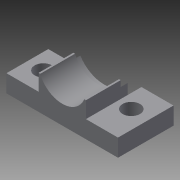
# Autodesk Inventor part: Gbase 3
Saved by Autodesk Inventor 2013 (Build 170138000, 138)
## iProperties
Created: 2016-06-22
Part Number: Gbase 3
Material: Generic
Document SubType Name: Modeling
Designer: labuser
Density: 1 g/cm^3
Author: labuser
Autodesk Inventor part; units mm, degrees
ref_plane "YZ Plane" through (0, 0, 0) normal (1, 0, 0) x (0, 1, 0)
ref_plane "XZ Plane" through (0, 0, 0) normal (0, 1, 0) x (-1, 0, 0)
ref_plane "XY Plane" through (0, 0, 0) normal (0, 0, 1) x (1, 0, 0)
sketch "Sketch1" plane through (0, 0, 0) normal (0, 1, 0) x (-1, 0, 0)
  line L0 (0, 0) -> (20.32, 0)
  line L1 (20.32, 0) -> (20.32, 7.62)
  line L2 (20.32, 7.62) -> (0, 7.62)
  line L3 (0, 7.62) -> (0, 0)
  dimension "d0" = 20.32
  dimension "d1" = 7.62
  constraints: 8 end point, 2 parallel, 1 horizontal, 1 perpendicular
  measures "d0" distance of L2.end L1.end
  measures "d1" distance of L1.end L0.end
extrude "Extrusion1" add sketch "Sketch1" along normal blind 3.175
sketch "Sketch2" plane through (0, 3.175, 0) normal (0, 1, 0) x (1, 0, 0)
  line L0 (0, 0) -> (-20.32, 0) projected
  line L1 (-20.32, 0) -> (-20.32, -7.62) projected
  line L2 (-20.32, -7.62) -> (0, -7.62) projected
  line L3 (-14.478, -7.62) -> (-5.842, -7.62)
  line L4 (-5.842, -7.62) -> (-5.842, 0)
  line L5 (-5.842, 0) -> (-14.478, 0)
  line L6 (-14.478, 0) -> (-14.478, -7.62)
  dimension "d4" = 8.636
  dimension "d5" = 5.842
  constraints: 8 end point, 2 parallel, 2 point on line, 1 horizontal, 1 perpendicular
  measures "d4" distance of L5.end L4.end
  measures "d5" distance between parallel lines of L6 L1
extrude "Extrusion2" add sketch "Sketch2" along normal blind 7.112 contours L4 L2 L6 L0
sketch "Sketch3" plane through (-20.32, 0, 7.62) normal (0, 0, 1) x (1, 0, 0)
  line L0 (14.478, 3.175) -> (14.478, 10.287) projected
  line L1 (5.842, 10.287) -> (14.478, 10.287) projected
  circle A0 centre (10.16, 7.747) radius 4.318
  line L2 (5.842, 10.287) -> (14.478, 10.287)
  line L3 (14.478, 10.287) -> (14.478, 7.747)
  line L4 (14.478, 7.747) -> (5.842, 7.747)
  line L5 (5.842, 7.747) -> (5.842, 10.287)
  line L6 (5.842, 7.747) -> (14.478, 7.747)
  line L7 (14.478, 7.747) -> (14.478, 6.1492)
  line L8 (14.478, 6.1492) -> (5.842, 6.1492)
  line L9 (5.842, 6.1492) -> (5.842, 7.747)
  dimension "d8" = 8.636
  dimension "d9" = 2.54
  constraints: 16 end point, 4 parallel, 2 horizontal, 2 perpendicular, 2 point on line, 1 horizontal alignment, 2 other
  measures "d9" distance from line of L1 point (10.16, 7.747)
extrude "Extrusion3" cut sketch "Sketch3" against normal up to surface (7.62 mm away)
sketch "Sketch5" plane through (0, 0, 0) normal (0, 0, -1) x (-1, 0, 0)
  arc A0 (6.1485, 6.1492) -> (14.1715, 6.1492) centre (10.16, 7.747) ccw projected
  circle A1 centre (10.16, 7.747) radius 5.08
  dimension "d21" = 10.16
  constraints: 1 centre point, 1 coincident
  measures "d21" diameter of A1
extrude "Extrusion5" cut sketch "Sketch5" against normal blind 1.27
sketch "Sketch4" plane through (0, 0, 0) normal (0, -1, 0) x (1, 0, 0)
  line L0 (-20.32, 7.62) -> (0, 7.62) projected
  line L1 (-20.32, 0) -> (-20.32, 7.62) projected
  circle A0 centre (-17.399, 3.81) radius 1.5875
  circle A1 centre (-3.302, 1.8923) radius 1.5875
  dimension "d12" = 3.175
  dimension "d14" = 3.81
  dimension "d15" = 2.921
  dimension "d16" = 3.175
  dimension "d26" = 14.097
  dimension "d27" = 1.9177
  constraints: 2 centre point
  measures "d12" diameter of A0
  measures "d14" distance from line of L0 A0.centre
  measures "d15" distance from line of L1 A0.centre
  measures "d16" diameter of A1
  measures "d26" horizontal distance of A0.centre A1.centre
  measures "d27" vertical distance of A0.centre A1.centre
extrude "Extrusion4" cut sketch "Sketch4" against normal up to next
sketch "Sketch6" plane through (0, 0, 0) normal (0, 0, -1) x (-1, 0, 0)
  line L0 (5.842, 3.175) -> (0, 3.175)
  line L1 (0, 3.175) -> (0, 0)
  line L2 (0, 0) -> (5.842, 0)
  line L3 (5.842, 0) -> (5.842, 3.175)
  constraints: 8 end point, 2 parallel, 1 horizontal, 1 perpendicular
extrude "Extrusion6" add sketch "Sketch6" along normal blind 2.5
body "Solid1"
